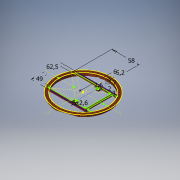
# Autodesk Inventor part: ODroid Holder-40x
Saved by Autodesk Inventor 2018 (Build 220112000, 112)
## iProperties
Part Number: ODroid Holder-40x
Material: Kupfer, Guss
Document SubType Name: Modeling
Designer: Jochen Alt
Mass: 179.761 g
Surface Area: 193.281 cm^2
Volume: 20.1075 cm^3
Density: 8.94 g/cm^3
Appearance: Kupfer - satiniert
Author: Jochen Alt
Autodesk Inventor part; units mm, degrees
ref_plane "YZ Plane" through (0, 0, 0) normal (1, 0, 0) x (0, 1, 0)
ref_plane "XZ Plane" through (0, 0, 0) normal (0, 1, 0) x (-1, 0, 0)
sketch "Skizze1" plane through (0, 0, 0) normal (0, 0, 1) x (1, 0, 0)
  circle A0 centre (0, 0) radius 59.3
  circle A1 centre (0, 0) radius 52.5
  circle A2 centre (0, 0) radius 53.6 construction
  line L0 (-83.17, 0) -> (83.92, 0) construction
  line L1 (35.006, -44.9842) -> (-1.8793, -56.969)
  line L2 (-54.7615, 15.817) -> (-31.9651, 47.1935)
  line L3 (-1.8793, 56.969) -> (35.006, 44.9842)
  line L4 (-31.9651, -47.1935) -> (-54.7615, -15.817)
  arc A3 (-31.9651, -47.1935) -> (-1.8793, -56.969) centre (0, 0) ccw
  arc A4 (-54.7615, 15.817) -> (-54.7615, -15.817) centre (0, 0) ccw
  arc A5 (35.006, -44.9842) -> (35.006, 44.9842) centre (0, 0) ccw
  arc A6 (-1.8793, 56.969) -> (-31.9651, 47.1935) centre (0, 0) ccw
  circle A7 centre (0, 0) radius 46.4646
  line L5 (16.5633, -50.9766) -> (0, 0) construction
  line L6 (0, 0) -> (-43.3633, -31.5053) construction
  line L7 (0, 0) -> (16.5633, 50.9766) construction
  line L8 (0, 0) -> (-43.3633, 31.5053) construction
  point P0 (60.05, 0)
  dimension "d7" = 118.6
  dimension "d100" = 105
  dimension "d108" = 107.2
  dimension "d110" = 57
  dimension "d115" = 6.0354
  dimension "d139" = 72
  dimension "d140" = 72
  dimension "d141" = 72
  dimension "d142" = 72
  constraints: 16 end point, 8 centre point, 8 point on circle, 6 coincident, 4 midpoint, 4 perpendicular, 3 concentric, 3 tangent, 2 other
  measures "d7" diameter of A0
  measures "d100" diameter of A1
  measures "d108" diameter of A2
  measures "d110" radius of A5
  measures "d115" radial gap between concentric circles of A7 A1
  measures "d139" angle of L5 L0
  measures "d140" angle of L0 L7
  measures "d141" angle of L7 L8
  measures "d142" angle of L6 L5
extrude "Extrusion3" add sketch "Skizze1" against normal blind 5 contours L1 A3 L4 A4 L2 A6 L3 A5
extrude "Extrusion4" add sketch "Skizze1" along normal blind 1.5 contours A0 | L1 A3 L4 A4 L2 A6 L3 A5
sketch "ODroidskizze" plane through (0, 0, 1.5) normal (0, 0, 1) x (1, 0, 0)
  line L0 (0, -83.02) -> (0, 83.02) construction
  line L1 (-83.02, 0) -> (83.02, 0) construction
  line L2 (8.7, -24.5009) -> (-49.3, -24.5009) construction
  line L3 (-49.3, -24.5009) -> (-49.3, 24.4991) construction
  line L4 (-49.3, 24.4991) -> (8.7, 24.4991) construction
  line L5 (8.7, 24.4991) -> (8.7, -24.5009) construction
  line L6 (8.7, -24.5009) -> (-49.3, 24.4991) construction
  line L7 (32.7, 28.25) -> (32.7, -28.25) construction
  line L8 (32.7, -28.25) -> (-53.1757, 34.4371) construction
  line L9 (-53.1757, -34.4371) -> (32.7, 28.25) construction
  line L10 (32.7, 26.253) -> (32.7, -26.25)
  line L11 (7.2, 20.7483) -> (10.2, 20.7483)
  line L12 (12.2, 22.7483) -> (12.2, 28.25)
  line L13 (5.2, 28.25) -> (5.2, 22.7483)
  line L14 (5.2, 20.7483) -> (12.2, 28.25) construction
  line L15 (12.2, 20.7483) -> (5.2, 28.25) construction
  line L16 (7.2, -20.7517) -> (10.2, -20.7517)
  line L17 (12.2, -22.7517) -> (12.2, -28.25)
  line L18 (5.2, -28.25) -> (5.2, -22.7517)
  line L19 (5.2, -20.7517) -> (12.2, -28.25) construction
  line L20 (12.2, -20.7517) -> (5.2, -28.25) construction
  arc A0 (5.2, 22.7483) -> (7.2, 20.7483) centre (7.2, 22.7483) ccw
  arc A1 (10.2, 20.7483) -> (12.2, 22.7483) centre (10.2, 22.7483) ccw
  arc A2 (12.2, -22.7517) -> (10.2, -20.7517) centre (10.2, -22.7517) ccw
  arc A3 (7.2, -20.7517) -> (5.2, -22.7517) centre (7.2, -22.7517) ccw
  arc A4 (32.7, 26.253) -> (30.7, 28.25) centre (30.7, 26.25) ccw
  arc A5 (30.7, -28.25) -> (32.7, -26.25) centre (30.7, -26.25) ccw
  line L21 (12.2, 28.25) -> (30.7, 28.25)
  line L22 (12.2, 28.25) -> (32.7, 28.25) construction
  line L23 (30.7, -28.25) -> (12.2, -28.25)
  line L24 (32.7, -28.25) -> (12.2, -28.25) construction
  circle A6 centre (0, 0) radius 59.3 projected
  line L25 (-42.1863, 31.25) -> (42.1863, 31.25)
  line L26 (-42.1863, -31.25) -> (42.1863, -31.25)
  line L27 (35.7, -26.25) -> (35.7, 26.25)
  line L28 (37.7, 28.25) -> (44.2514, 28.25)
  line L29 (44.2514, -28.25) -> (37.7, -28.25)
  arc A7 (37.7, 28.25) -> (35.7, 26.25) centre (37.7, 26.25) ccw
  arc A8 (35.7, -26.25) -> (37.7, -28.25) centre (37.7, -26.25) ccw
  circle A9 centre (8.7, 24.4991) radius 1.3
  circle A10 centre (8.7, -24.5009) radius 1.3
  circle A11 centre (0, 0) radius 52.5 projected
  line L30 (-44.2514, 28.25) -> (5.2, 28.25) construction
  line L31 (-44.2514, 28.25) -> (5.2, 28.25)
  line L32 (5.2, -28.25) -> (-44.2514, -28.25)
  line L33 (5.2, -28.25) -> (-44.2514, -28.25) construction
  point P0 (0.9483, -27.9891)
  point P1 (-20.301, 0)
  point P2 (-20.301, 0)
  point P3 (-6, 0)
  point P4 (44.0485, 0)
  point P5 (-44.8148, -28.2558)
  point P6 (44.8435, -28.25)
  point P7 (44.8435, 28.25)
  point P8 (-44.8435, -28.25)
  point P9 (53, 0)
  point P10 (-53.0251, 0)
  dimension "d30" = 49
  dimension "d31" = 58
  dimension "d38" = 6
  dimension "d39" = 7
  dimension "d40" = 7
  dimension "d69" = 3
  dimension "d70" = 2
  dimension "d114" = 5.2
  dimension "d134" = 62.5
  dimension "d135" = 2.6
  dimension "d136" = 2.6
  constraints: 64 end point, 17 tangent, 16 point on circle, 15 point on line, 13 parallel, 10 centre point, 10 horizontal, 7 coincident, 6 perpendicular, 5 equal radius, 4 midpoint, 2 collinear, 11 other
  measures "d30" distance between parallel lines of L2 L4
  measures "d31" distance between parallel lines of L5 L3
  measures "d38" distance from line of L0 point (-6, 0)
  measures "d39" distance between parallel lines of L12 L13
  measures "d40" distance between parallel lines of L17 L18
  measures "d69" distance between parallel lines of L27 L10
  measures "d70" radius of A7
  measures "d114" distance between parallel lines of L13 L0
  measures "d134" distance between parallel lines of L25 L26
  measures "d135" diameter of A9
  measures "d136" diameter of A10
extrude "Extrusion5" add sketch "ODroidskizze" against normal blind 3.5 contours A4 L21 L12 A1 L11 A0 L13 L31 A11 L25 L28 A7 L27 A8 L29 L26 L32 L18 A3 L16 A2 L17 L23 A5 L10
ref_plane "Arbeitsebene1" through (0, 0, -1) normal (0, 0, 1) x (1, 0, 0)
sketch "Skizze8" plane through (0, 0, 1.5) normal (0, 0, 1) x (1, 0, 0)
  arc A0 (42.1863, 31.25) -> (-42.1863, 31.25) centre (0, 0) ccw construction
  arc A1 (-42.1863, -31.25) -> (42.1863, -31.25) centre (0, 0) ccw construction
  circle A2 centre (-17.9561, -49.3339) radius 2
  circle A3 centre (-17.9561, 49.3339) radius 2
  line L0 (-83.02, 0) -> (83.02, 0) construction
  line L1 (-17.9561, -49.3339) -> (0, 0) construction
  line L2 (0, 0) -> (-17.9561, 49.3339) construction
  dimension "d116" = 4
  dimension "d117" = 4
  dimension "d143" = 70
  dimension "d144" = 70
  constraints: 4 end point, 4 point on circle, 2 centre point
  measures "d116" diameter of A2
  measures "d117" diameter of A3
  measures "d143" angle of L0 L1
  measures "d144" angle of L0 L2
extrude "Lidar-Holder-Nose" cut sketch "Skizze8" against normal up to next
chamfer "Fase5" distance 0.5 angle 45 14 edges at (-43.3633, -31.5053, -5) (-57, 0, -5) (-17.614, -54.2102, -5) (-43.3633, 31.5053, -5) (-17.614, 54.2102, -5) (16.5633, 50.9766, -5) (57, 0, -5) (16.5633, -50.9766, -5) (-32.1969, -41.4682, 1.5) (16.0722, -49.9793, 1.5) (16.0722, 49.9793, 1.5) (-32.1969, 41.4682, 1.5) (-18.6401, 51.2132, 1.5) (-18.6401, -51.2132, 1.5)
fillet "Rundung4" radius 2 8 edges at (-44.2514, -28.25, -0.25) (44.2514, -28.25, -0.25) (44.2514, 28.25, -0.25) (-44.2514, 28.25, -0.25) (12.2, 28.25, -0.25) (5.2, 28.25, -0.25) (5.2, -28.25, -0.25) (12.2, -28.25, -0.25)
